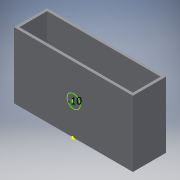
# Autodesk Inventor part: Bevel holder
Saved by Autodesk Inventor 2019 (Build 230136000, 136)
## iProperties
Created: 2019-10-27
Part Number: Bevel holder
Material: Generic
Document SubType Name: Modeling
Designer: Mark
Density: 1 g/cm^3
Appearance: Default
Author: Mark
Autodesk Inventor part; units mm, degrees
ref_plane "YZ Plane" through (0, 0, 0) normal (1, 0, 0) x (0, 1, 0)
ref_plane "XZ Plane" through (0, 0, 0) normal (0, 1, 0) x (-1, 0, 0)
ref_plane "XY Plane" through (0, 0, 0) normal (0, 0, 1) x (1, 0, 0)
sketch "Sketch1" plane through (0, 0, 0) normal (0, 1, 0) x (-1, 0, 0)
  line L0 (45, 12.5) -> (-45, 12.5)
  line L1 (-45, 12.5) -> (-45, -12.5)
  line L2 (-45, -12.5) -> (45, -12.5)
  line L3 (45, -12.5) -> (45, 12.5)
  line L4 (45, 12.5) -> (-45, -12.5) construction
  line L5 (-45, 12.5) -> (45, -12.5) construction
  line L6 (43, 10.5) -> (-43, 10.5)
  line L7 (-43, 10.5) -> (-43, -10.5)
  line L8 (-43, -10.5) -> (43, -10.5)
  line L9 (43, -10.5) -> (43, 10.5)
  line L10 (43, 10.5) -> (-43, -10.5) construction
  line L11 (-43, 10.5) -> (43, -10.5) construction
  point P0 (0, 0)
  dimension "d0" = 90
  dimension "d1" = 25
  dimension "d2" = 86
  dimension "d3" = 21
  constraints: 24 end point, 4 midpoint, 4 parallel, 2 horizontal, 2 perpendicular
  measures "d0" distance of L2.end L1.end
  measures "d1" distance of L1.end L0.end
  measures "d2" distance of L8.end L7.end
  measures "d3" distance of L7.end L6.end
extrude "Extrusion1" add sketch "Sketch1" along normal blind 50
sketch "Sketch2" plane through (-45, 0, 12.5) normal (0, 0, 1) x (1, 0, 0)
  circle A0 centre (45, 25) radius 9.65
  line L0 (90, 0) -> (90, 50) projected
  line L1 (0, 50) -> (90, 50) projected
  point P0 (45, 0)
  dimension "d6" = 19.3
  dimension "d7" = 45
  dimension "d8" = 25
  constraints: 1 centre point
  measures "d6" diameter of A0
  measures "d7" distance from line of L0 A0.centre
  measures "d8" distance from line of L1 A0.centre
extrude "Extrusion2" cut sketch "Sketch2" against normal blind 29.05
sketch "Sketch3" plane through (45, 0, 12.5) normal (1, 0, 0) x (0, 0, -1)
  circle A0 centre (19.5, 10) radius 2.65
  circle A1 centre (5.5, 10) radius 2.65
  circle A2 centre (19.5, 40) radius 2.65
  circle A3 centre (5.5, 40) radius 2.65
  line L0 (0, 50) -> (25, 50) projected
  line L1 (25, 0) -> (25, 50) projected
  line L2 (0, 0) -> (0, 50) projected
  line L3 (0, 0) -> (25, 0) projected
  point P0 (12.5, 0)
  dimension "d11" = 5.3
  dimension "d12" = 5.3
  dimension "d13" = 5.3
  dimension "d14" = 5.3
  dimension "d15" = 10
  dimension "d16" = 10
  dimension "d17" = 5.5
  dimension "d18" = 5.5
  dimension "d19" = 10
  dimension "d20" = 5.5
  dimension "d21" = 5.5
  dimension "d22" = 10
  constraints: 4 centre point
  measures "d11" diameter of A0
  measures "d12" diameter of A1
  measures "d13" diameter of A2
  measures "d14" diameter of A3
  measures "d15" distance from line of L0 A3.centre
  measures "d16" distance from line of L0 A2.centre
  measures "d17" distance from line of L1 A2.centre
  measures "d18" distance from line of L2 A3.centre
  measures "d19" distance from line of L3 A1.centre
  measures "d20" distance from line of L2 A1.centre
  measures "d21" distance from line of L1 A0.centre
  measures "d22" distance from line of L3 A0.centre
extrude "Extrusion3" cut sketch "Sketch3" against normal blind 143.35 contours A0 | A1 | A2 | A3
body "Solid1"
